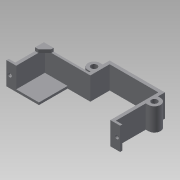
# Autodesk Inventor part: センサ冶具2個積み左
Saved by Autodesk Inventor 2017 (Build 210142000, 142)
## iProperties
Part Number: センサ冶具2個積み左
Material: 一般
Document SubType Name: Modeling
Designer: HISAAKI
Density: 1 g/cm^3
Appearance: 既定
Author: HISAAKI
Autodesk Inventor part; units mm, degrees
ref_plane "YZ Plane" through (0, 0, 0) normal (1, 0, 0) x (0, 1, 0)
ref_plane "XZ Plane" through (0, 0, 0) normal (0, 1, 0) x (-1, 0, 0)
ref_plane "XY Plane" through (0, 0, 0) normal (0, 0, 1) x (1, 0, 0)
sketch "スケッチ1" plane through (0, 0, 0) normal (0, 0, 1) x (1, 0, 0)
  line L0 (0, 0) -> (0, 17.65)
  line L1 (0, 17.65) -> (28, 17.65)
  line L2 (28, 17.65) -> (28, 30.15)
  line L3 (28, 30.15) -> (58, 30.15)
  line L4 (58, 30.15) -> (58, 0)
  line L5 (58, 0) -> (60, 0)
  line L6 (60, 0) -> (60, 32.15)
  line L7 (60, 32.15) -> (28, 32.15)
  line L8 (28, 32.15) -> (26, 32.15)
  line L9 (26, 32.15) -> (26, 19.65)
  line L10 (26, 19.65) -> (-2, 19.65)
  line L11 (-2, 19.65) -> (-2, 0)
  line L12 (-2, 0) -> (0, 0)
  dimension "d0" = 17.65
  dimension "d1" = 28
  dimension "d2" = 12.5
  dimension "d3" = 30
  dimension "d4" = 2
  dimension "d5" = 32.15
  dimension "d6" = 32
  dimension "d7" = 2
  dimension "d8" = 12.5
  dimension "d9" = 28
  constraints: 26 end point, 7 perpendicular, 3 parallel, 3 point on line, 1 vertical
  measures "d0" distance of L0.start L0.end
  measures "d1" distance of L0.end L1.end
  measures "d2" distance of L1.end L2.end
  measures "d3" distance of L2.end L3.end
  measures "d4" distance of L4.end L5.end
  measures "d5" distance of L5.end L6.end
  measures "d6" distance of L6.end L7.end
  measures "d7" distance of L7.end L8.end
  measures "d8" distance of L8.end L9.end
  measures "d9" distance of L9.end L10.end
extrude "押し出し1" add sketch "スケッチ1" along normal blind 14
sketch "スケッチ2" plane through (60, 0, 0) normal (1, 0, 0) x (0, 0, -1)
  line L0 (0, 0) -> (-14, 0) projected
  line L1 (-14, 0) -> (0, 0)
  line L2 (0, 0) -> (0, 2)
  line L3 (0, 2) -> (-14, 2)
  line L4 (-14, 2) -> (-14, 0)
  dimension "d12" = 14
  dimension "d13" = 2
  constraints: 8 end point, 2 parallel, 1 horizontal, 1 perpendicular
  measures "d12" distance of L3.end L2.end
  measures "d13" distance of L2.end L1.end
extrude "押し出し2" add sketch "スケッチ2" along normal blind 7
sketch "スケッチ3" plane through (-2, 0, 0) normal (-1, 0, 0) x (0, 0, 1)
  line L0 (14, 2) -> (0, 2) projected
  line L1 (0, 0) -> (14, 0)
  line L2 (14, 0) -> (14, 2)
  line L3 (14, 2) -> (0, 2)
  line L4 (0, 2) -> (0, 0)
  dimension "d16" = 14
  constraints: 8 end point, 2 parallel, 1 horizontal, 1 perpendicular
  measures "d16" distance of L3.end L0.start
extrude "押し出し3" add sketch "スケッチ3" along normal blind 7
sketch "スケッチ4" plane through (0, 0, 14) normal (0, 0, 1) x (1, 0, 0)
  line L0 (60, 32.15) -> (60, 24.15)
  line L1 (60, 24.15) -> (61.6, 24.15)
  arc A0 (61.6, 20.4) -> (61.6, 27.9) centre (61.6, 24.15) ccw
  line L2 (61.6, 24.15) -> (61.6, 20.4) construction
  line L3 (61.6, 24.15) -> (61.6, 27.9) construction
  line L4 (61.6, 27.9) -> (60, 27.9)
  line L5 (61.6, 20.4) -> (60, 20.4)
  line L6 (60, 2) -> (60, 32.15) projected
  line L7 (60, 27.9) -> (60, 20.4)
  point P0 (0, 0)
  dimension "d47" = 8
  dimension "d48" = 1.6
  dimension "d49" = 3.75
  dimension "d50" = 180
  constraints: 14 end point, 2 perpendicular, 2 point on circle, 2 point on line, 1 centre point, 1 coincident, 1 horizontal, 1 parallel, 1 vertical
  measures "d47" distance of L0.start L0.end
  measures "d48" distance of L0.end L1.end
  measures "d49" radius of A0
  measures "d50" angle of L3 L2
extrude "押し出し4" add sketch "スケッチ4" against normal blind 14
hole "穴3" at (61.6, 24.15, 14) direction (0, 0, -1) diameter 3.75 end through all
sketch "スケッチ7" plane through (0, 0, 14) normal (0, 0, 1) x (1, 0, 0)
  line L0 (60, 32.15) -> (26, 32.15) projected
  line L1 (26, 32.15) -> (26, 24.15)
  line L2 (26, 24.15) -> (24.4, 24.15)
  arc A0 (24.4, 27.9) -> (24.4, 20.4) centre (24.4, 24.15) ccw
  line L3 (24.4, 27.9) -> (26, 27.9)
  line L4 (24.4, 20.4) -> (26, 20.4)
  line L5 (26, 20.4) -> (26, 27.9)
  line L6 (26, 32.15) -> (26, 19.65) projected
  circle A1 centre (24.4, 24.15) radius 1.875
  point P0 (0, 0)
  dimension "d60" = 8
  dimension "d61" = 1.6
  dimension "d62" = 3.75
  dimension "d63" = 3.75
  constraints: 10 end point, 2 centre point, 2 coincident, 2 perpendicular, 2 point on circle, 1 collinear, 1 horizontal, 1 point on line, 1 vertical
  measures "d60" distance of L0.end L1.end
  measures "d61" distance of L1.end L2.end
  measures "d62" radius of A0
  measures "d63" diameter of A1
extrude "押し出し6" add sketch "スケッチ7" against normal blind 14 contours L1 A1 L5 L4 A0 L3 | L1 L5 A1 picked at (23.6929, 24.15)
hole "穴4" at (24.4, 24.15, 14) direction (0, 0, -1) diameter 3.75 end through all
sketch "スケッチ10" plane through (0, 17.65, 0) normal (0, -1, 0) x (1, 0, 0)
  line L0 (28, 14) -> (58, 14) projected
  line L1 (0, 0) -> (28, 0)
  line L2 (28, 0) -> (28, 14)
  line L3 (28, 14) -> (0, 14)
  line L4 (0, 14) -> (0, 0)
  constraints: 8 end point, 2 parallel, 1 horizontal, 1 perpendicular
extrude "押し出し7" cut sketch "スケッチ10" against normal blind 0.6
sketch "スケッチ11" plane through (0, 0, 0) normal (0, -1, 0) x (1, 0, 0)
  line L0 (0, 14) -> (-9, 14) projected
  line L1 (60, 0) -> (67, 0) projected
  line L2 (-9, 14) -> (67, 14)
  line L3 (67, 14) -> (67, 0)
  line L4 (67, 0) -> (-9, 0)
  line L5 (-9, 0) -> (-9, 14)
  point P0 (0, 0)
  constraints: 8 end point, 2 parallel, 1 horizontal, 1 perpendicular
extrude "押し出し8" cut sketch "スケッチ11" against normal blind 0.6
sketch "スケッチ12" plane through (0, 0, 14) normal (0, 0, 1) x (1, 0, 0)
  line L0 (-2, 19.65) -> (-2, 2) projected
  line L1 (-2, 19.65) -> (4, 19.65)
  line L2 (26, 19.65) -> (-2, 19.65) projected
  line L3 (4, 19.65) -> (4, 18.25)
  line L4 (0, 18.25) -> (28, 18.25) projected
  line L5 (4, 18.25) -> (0.2844, 14.5344)
  line L6 (4, 18.25) -> (9.2547, 18.25) construction
  line L7 (0.2844, 14.5344) -> (0, 14.25)
  line L8 (0, 0.6) -> (0, 18.25) projected
  line L9 (0, 14.25) -> (-2, 14.25)
  line L10 (-2, 14.25) -> (-2, 19.65)
  point P0 (0, 0)
  dimension "d79" = 6
  dimension "d80" = 135
  constraints: 14 end point, 4 point on line, 2 horizontal, 2 perpendicular, 1 equal length
  measures "d79" distance of L0.start L1.end
  measures "d80" angle of L5 L6
extrude "押し出し9" add sketch "スケッチ12" along normal blind 2
sketch "スケッチ15" plane through (0, 0, 0) normal (0, 0, -1) x (-1, 0, 0)
  line L0 (0, 0.6) -> (0, 18.25) projected
  line L1 (0, 18.25) -> (-14, 18.25)
  line L2 (-14, 18.25) -> (-14, 0.6)
  line L3 (-14, 0.6) -> (0, 0.6)
  line L4 (0, 0.6) -> (0, 18.25)
  point P0 (0, 0)
  dimension "d88" = 14
  constraints: 8 end point, 2 parallel, 1 horizontal, 1 perpendicular
  measures "d88" distance of L3.end L2.end
extrude "押し出し11" add sketch "スケッチ15" against normal blind 1.4
sketch "スケッチ17" plane through (67, 0, 0) normal (1, 0, 0) x (0, 0, -1)
  line L0 (0, 0.6) -> (-14, 0.6) projected
  line L1 (0, 0.6) -> (-14, 0.6)
  line L2 (-14, 0.6) -> (-14, 9.5309)
  line L3 (-14, 9.5309) -> (0, 9.5309)
  line L4 (0, 9.5309) -> (0, 0.6)
  point P0 (0, 0)
  constraints: 8 end point, 2 parallel, 1 horizontal, 1 perpendicular
extrude "押し出し13" cut sketch "スケッチ17" against normal blind 3
sketch "スケッチ18" plane through (-9, 0, 0) normal (-1, 0, 0) x (0, 0, 1)
  line L0 (0, 0.6) -> (14, 0.6) projected
  line L1 (0, 0.6) -> (14, 0.6)
  line L2 (14, 0.6) -> (14, 6.5)
  line L3 (14, 6.5) -> (0, 6.5)
  line L4 (0, 6.5) -> (0, 0.6)
  point P0 (0, 0)
  constraints: 8 end point, 2 parallel, 1 horizontal, 1 perpendicular
extrude "押し出し14" cut sketch "スケッチ18" against normal blind 3
hole "穴5" at (-4, 2, 7) direction (0, -1, 0) diameter 2.4 end through all
hole "穴6" at (62, 2, 7) direction (0, -1, 0) diameter 2.4 end through all
